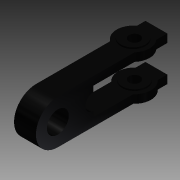
# Autodesk Inventor part: pulley hook
Saved by Autodesk Inventor 2014 (Build 180170000, 170)
## iProperties
Created: 2013-10-13
Part Number: pulley hook
Material: Acetal Resin, Black
Document SubType Name: Modeling
Designer: david
Density: 1.425 g/cm^3
Appearance: Smooth - Black
Author: david
Autodesk Inventor part; units mm, degrees
ref_plane "YZ Plane" through (0, 0, 0) normal (1, 0, 0) x (0, 1, 0)
ref_plane "XZ Plane" through (0, 0, 0) normal (0, 1, 0) x (-1, 0, 0)
ref_plane "XY Plane" through (0, 0, 0) normal (0, 0, 1) x (1, 0, 0)
sketch "Sketch1" plane through (0, 0, 0) normal (1, 0, 0) x (0, 1, 0)
  line L0 (0, 0.9489) -> (25.4, 0.9489)
  line L1 (25.4, 0.9489) -> (25.4, 77.1489)
  line L2 (25.4, 77.1489) -> (0, 77.1489)
  line L3 (0, 77.1489) -> (0, 0.9489)
  point P0 (0, 0)
  dimension "d0" = 25.4
  dimension "d1" = 76.2
  constraints: 8 end point, 2 parallel, 1 horizontal, 1 perpendicular
  measures "d0" distance of L0.start L0.end
  measures "d1" distance of L0.end L1.end
extrude "Extrusion1" add sketch "Sketch1" along normal blind 12.7
sketch "Sketch2" plane through (0, 0, 0) normal (-1, 0, 0) x (0, 0, 1)
  line L0 (77.1489, 25.4) -> (77.1489, 0) projected
  line L1 (0.9489, 25.4) -> (77.1489, 25.4) projected
  point P0 (0, 0)
  point P1 (64.4489, 12.7)
  dimension "d4" = 12.7
  dimension "d5" = 12.7
  measures "d4" distance from line of L0 point (64.449, 12.7)
  measures "d5" distance from line of L1 point (64.449, 12.7)
hole "Hole1" at (0, 12.7, 64.4489) direction (1, 0, 0) diameter 12.7 end through all
fillet "Fillet1" radius 12.7 2 edges at (6.35, 25.4, 77.1489) (6.35, 0, 77.1489)
sketch "Sketch3" plane through (0, 0, 0) normal (-1, 0, 0) x (0, 0, 1)
  line L0 (0.9489, 25.4) -> (64.4489, 25.4) projected
  line L1 (0.9489, 0) -> (0.9489, 25.4) projected
  line L2 (64.4489, 0) -> (0.9489, 0) projected
  line L3 (0.9489, 20.6375) -> (43.8114, 20.6375)
  line L4 (43.8114, 4.7625) -> (0.9489, 4.7625)
  line L5 (0.9489, 4.7625) -> (0.9489, 20.6375)
  arc A0 (43.8114, 7.9375) -> (43.8114, 17.4625) centre (43.8114, 12.7) ccw
  line L6 (43.8114, 20.6375) -> (43.8114, 17.4625)
  line L7 (43.8114, 7.9375) -> (43.8114, 4.7625)
  point P0 (0, 0)
  dimension "d15" = 4.7625
  dimension "d16" = 4.7625
  dimension "d18" = 3.175
  dimension "d19" = 3.175
  dimension "d20" = 4.7625
  dimension "d21" = 42.8625
  constraints: 10 end point, 2 perpendicular, 2 point on circle, 1 centre point, 1 horizontal, 1 parallel, 1 point on line
  measures "d15" distance between parallel lines of L0 L3
  measures "d16" distance between parallel lines of L2 L4
  measures "d18" distance of L3.end L6.end
  measures "d19" distance of L4.start L7.start
  measures "d20" radius of A0
  measures "d21" horizontal distance of A0.centre L3.start
extrude "Extrusion2" cut sketch "Sketch3" against normal through all
sketch "Sketch4" plane through (0, 0, 0.9489) normal (0, -1, 0) x (1, 0, 0)
  line L0 (0, 0) -> (12.7, 0) projected
  circle A0 centre (6.35, 12.7) radius 9.525
  line L1 (12.7, 63.5) -> (12.7, 0) projected
  point P0 (0, -0.9489)
  dimension "d24" = 12.7
  dimension "d25" = 19.05
  dimension "d49" = 6.35
  constraints: 1 centre point
  measures "d24" distance from line of L0 A0.centre
  measures "d25" diameter of A0
  measures "d49" distance from line of L1 A0.centre
extrude "Extrusion3" add sketch "Sketch4" along normal up to surface (4.7625 mm away) from surface at -4.7625
sketch "Sketch5" plane through (0, 25.4, 0.9489) normal (0, 1, 0) x (1, 0, 0)
  circle A0 centre (5.5563, -12.7) radius 9.525
  point P0 (12.7, 0)
  point P1 (0, 0.9489)
  dimension "d28" = 19.05
  dimension "d29" = 12.7
  constraints: 1 centre point
  measures "d28" diameter of A0
  measures "d29" vertical distance of point (12.7, 0) A0.centre
extrude "Extrusion4" add sketch "Sketch5" along normal up to surface (4.7625 mm away) from surface at -4.7625
sketch "Sketch6" plane through (0, 25.4, 0.9489) normal (0, 1, 0) x (1, 0, 0)
  arc A0 (12.7, -19.0002) -> (12.7, -6.3998) centre (5.5563, -12.7) ccw projected
  circle A1 centre (5.5563, -12.7) radius 7.1438
  point P0 (0, 0.9489)
  dimension "d32" = 14.2875
  constraints: 1 centre point, 1 coincident
  measures "d32" diameter of A1
extrude "Extrusion5" add sketch "Sketch6" along normal blind 0.7937 and the other way blind 5.5563
sketch "Sketch7" plane through (0, 0, 0.9489) normal (0, -1, 0) x (1, 0, 0)
  arc A0 (12.7, 5.6005) -> (12.7, 19.7995) centre (6.35, 12.7) ccw projected
  circle A1 centre (6.35, 12.7) radius 7.1437
  point P0 (0, -0.9489)
  dimension "d37" = 14.2875
  constraints: 1 centre point, 1 coincident
  measures "d37" diameter of A1
extrude "Extrusion6" add sketch "Sketch7" along normal blind 0.7937 and the other way blind 5.5563
sketch "Sketch8" plane through (6.35, -0.7938, 13.6489) normal (0, -1, 0) x (1, 0, 0)
  circle A0 centre (0, 0) radius 7.1437 projected
  point P0 (-6.35, -13.6489)
  constraints: 3 coincident
hole "Hole2" at (6.35, -0.7938, 13.6489) direction (0, 1, 0) diameter 6.35 end through all
body "Solid1"
